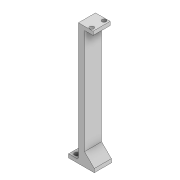
# Autodesk Inventor part: compass mount
Saved by Autodesk Inventor 2022 (Build 260153000, 153)
## iProperties
Created: 2024-08-29
Part Number: compass mount
Material: Generic
Document SubType Name: Modeling
Designer: david
Density: 1 g/cm^3
Appearance: Default
Author: david
Autodesk Inventor part; units mm, degrees
ref_plane "YZ Plane" through (0, 0, 0) normal (1, 0, 0) x (0, 1, 0)
ref_plane "XZ Plane" through (0, 0, 0) normal (0, 1, 0) x (-1, 0, 0)
ref_plane "XY Plane" through (0, 0, 0) normal (0, 0, 1) x (1, 0, 0)
sketch "Sketch1" plane through (0, 0, 0) normal (0, 0, 1) x (1, 0, 0)
  line L0 (-2.5, 100) -> (2.5, 100)
  line L1 (2.5, 100) -> (2.5, 0)
  line L2 (2.5, 0) -> (-2.5, 0)
  line L3 (-2.5, 0) -> (-2.5, 100)
  line L4 (0, -20) -> (0, 120) projected
  line L5 (-3.5, 0) -> (3.5, 0) projected
  point P0 (0, 0)
  point P1 (0, 100)
  dimension "d0" = 5
  dimension "d1" = 100
  constraints: 8 end point, 2 parallel, 1 collinear, 1 horizontal, 1 midpoint, 1 perpendicular, 1 vertical alignment
  measures "d0" distance of L0.start L0.end
  measures "d1" distance from line of L0 point (0, 0)
extrude "Extrusion1" add sketch "Sketch1" along normal mid plane 14
sketch "Sketch2" plane through (-2.5, 100, 7) normal (0, 1, 0) x (1, 0, 0)
  line L0 (5, 0) -> (0, 0) projected
  line L1 (0, 0) -> (12, 0)
  line L2 (12, 0) -> (12, 14)
  line L3 (12, 14) -> (0, 14)
  line L4 (0, 14) -> (0, 0)
  line L5 (0, 14) -> (5, 14) projected
  line L6 (5, 14) -> (5, 0) projected
  point P0 (2.5, 7)
  dimension "d5" = 7
  constraints: 8 end point, 2 parallel, 1 collinear, 1 horizontal, 1 perpendicular
  measures "d5" distance between parallel lines of L6 L2
extrude "Extrusion2" add sketch "Sketch2" against normal blind 3
sketch "Sketch3" plane through (-2.5, 100, 7) normal (0, 1, 0) x (1, 0, 0)
  line L0 (12, 0) -> (12, 14) projected
  line L1 (0, 14) -> (12, 14) projected
  line L2 (0, 0) -> (12, 0) projected
  point P0 (2.5, 7)
  point P1 (9, 2)
  point P2 (9, 12)
  dimension "d8" = 3
  dimension "d9" = 2
  dimension "d10" = 2
  constraints: 1 vertical alignment
  measures "d8" distance from line of L0 point (9, 12)
  measures "d9" distance from line of L1 point (9, 12)
  measures "d10" distance from line of L2 point (9, 2)
hole "Hole1" at (6.5, 100, 5) at (6.5, 100, -5) direction (0, -1, 0) diameter 3.4 end through all
sketch "Sketch4" plane through (-2.5, 0, 7) normal (0, -1, 0) x (1, 0, 0)
  line L0 (-8, 0) -> (13, 0)
  line L1 (13, 0) -> (13, -14)
  line L2 (13, -14) -> (-8, -14)
  line L3 (-8, -14) -> (-8, 0)
  line L4 (0, 0) -> (5, 0) projected
  line L5 (5, -14) -> (0, -14) projected
  line L6 (0, -14) -> (0, 0) projected
  line L7 (12, -14) -> (12, 0) projected
  line L8 (5, 0) -> (5, -14) projected
  point P0 (2.5, -7)
  dimension "d18" = 8
  dimension "d20" = 8
  constraints: 8 end point, 2 collinear, 2 parallel, 1 horizontal, 1 perpendicular
  measures "d18" distance between parallel lines of L3 L6
  measures "d20" distance between parallel lines of L8 L1
extrude "Extrusion3" add sketch "Sketch4" against normal blind 3
sketch "Sketch5" plane through (-2.5, 3, 7) normal (0, 1, 0) x (1, 0, 0)
  line L0 (-4.5, 11) -> (-4.5, 3) construction
  line L1 (-8, 14) -> (-8, 0) construction
  point P0 (2.5, 7)
  point P1 (-4.5, 7)
  point P2 (-8, 7)
  dimension "d23" = 8
  dimension "d24" = 3.5
  constraints: 2 end point, 2 midpoint, 1 horizontal alignment, 1 vertical, 1 vertical alignment
  measures "d23" distance of L0.end L0.start
  measures "d24" distance from line of L1 L0.start
hole "Hole2" at (-7, 3, -4) at (-7, 3, 4) direction (0, -1, 0) diameter 3.4 end through all
chamfer "Chamfer1" distance 8 angle 45 1 edges at (2.5, 3, 0)
chamfer "Chamfer2" distance 1 angle 45 1 edges at (-2.5, 3, 0)
equation "\"d10\" = d9"
body "Solid1"
